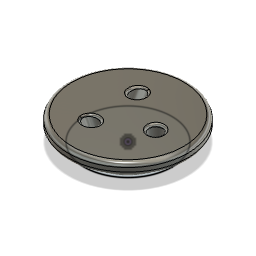
tappo (Autodesk Fusion 360 design; units mm, degrees)
Autodesk Fusion 360 part; units mm, degrees
sketch "Schizzo1" plane through (0, 0, 0) normal (0, 1, 0) x (1, 0, 0)
  circle A0 centre (0, 0) radius 11.05
  dimension "d1" = 22.1
  constraint coincident A0.centre origin
  measures "d1" diameter of A0
extrude "Estrusione1" add sketch "Schizzo1" along normal blind 3
sketch "Schizzo2" plane through (0, 3, 0) normal (0, 1, 0) x (-1, 0, 0)
  circle A0 centre (0, 0) radius 11.05
  circle A1 centre (0, 0) radius 15.05
  dimension "d4" = 4
  constraint coincident A0.centre A1.centre
  measures "d4" distance of A0 A1
extrude "Estrusione2" add sketch "Schizzo2" along normal blind 3 contours A0 | A1
fillet "Raccordo1" radius 1 3 edges at (14.0315, 6, -5.4423) (14.0315, 3, -5.4423) (-10.3022, 0, 3.9959)
fillet "Raccordo2" radius 0.5 1 edges at (-10.3022, 3, 3.9959)
ref_plane "Piano di lavoro1" through (0, 4.6647, 13.1079) normal (0, -0.335274, -0.942121) x (1, 0, 0)
sketch "Schizzo4" plane through (0, 6, 0) normal (0, 1, 0) x (-1, 0, 0)
  circle A0 centre (0, 0) radius 14.05
  circle A1 centre (-7, 0) radius 1.6
  line L0 (0, 0) -> (-11, 0)
  line L1 (0, 0) -> (5.674, -9.8276)
  line L2 (0, 0) -> (5.674, 9.8276)
  circle A2 centre (3.5, -6.0622) radius 1.6
  circle A3 centre (3.5, 6.0622) radius 1.6
  dimension "d12" = 3.2
  dimension "d13" = 120
  dimension "d14" = 120
  constraint coincident A0.centre L0.start
  constraint horizontal L0
  constraint symmetric A1 L2 A2
  constraint symmetric A1 L1 A3
  measures "d12" diameter of A1
  measures "d13" angle of L0 L1
  measures "d14" angle of L1 L2
ref_plane "Piano di lavoro3" through (-4.0972, 5.9367, 13.0728) normal (0.104736, 0.936674, -0.334174) x (-0.993806, 0.111125, 0)
ref_plane "Piano di lavoro4" through (-1.5836, 28.4168, 5.0526) normal (0.104736, 0.936674, -0.334174) x (-0.993806, 0.111125, 0)
hole "Foratura1" at (-1.6427, 22.361, -11.9401) direction (-0.104736, -0.936674, 0.334174) diameter 3.4 depth 27 tip angle 118
pattern_circular "Serie C1" count 3 over 240 about axis through (0, 3.5, 0) along (0, 1, 0) both ways of "Foratura1"
fillet "Raccordo3" radius 0.5 3 edges at (8.2499, 6, 1.3806) (-5.3206, 6, 6.4543) (-2.9293, 6, -7.8349)
